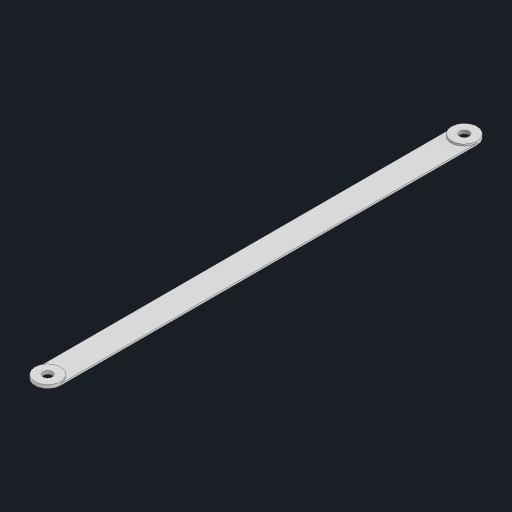
# Autodesk Inventor part: kozepso szalag2
Saved by Autodesk Inventor 2023 (Build 270158000, 158)
## iProperties
Created: 2022-11-11
Part Number: kozepso szalag2
Material: Generic
Document SubType Name: Modeling
Designer: gd1
Density: 1 g/cm^3
Appearance: Default
Mass: 4.10146 g
Surface Area: 82.9042 cm^2
Volume: 4.10146 cm^3
Author: gd1
Autodesk Inventor part; units mm, degrees
ref_plane "YZ Plane" through (0, 0, 0) normal (1, 0, 0) x (0, 1, 0)
ref_plane "XZ Plane" through (0, 0, 0) normal (0, 1, 0) x (-1, 0, 0)
ref_plane "XY Plane" through (0, 0, 0) normal (0, 0, 1) x (1, 0, 0)
sketch "Sketch1" plane through (0, 0, 0) normal (0, 1, 0) x (-1, 0, 0)
  circle A0 centre (0, 0) radius 2.75
  circle A1 centre (0, 0) radius 7.5
  circle A2 centre (0, -244.423) radius 2.75
  circle A3 centre (0, -244.423) radius 7.5
  line L0 (0, 7.5) -> (0, -251.923) construction
  line L1 (7.5, 0) -> (7.5, -244.423)
  line L2 (-7.5, 0) -> (-7.5, -244.423)
  dimension "d0" = 5.5
  dimension "d1" = 15
  dimension "d14" = 5.5
  dimension "d15" = 15
  dimension "d20" = 259.423
  constraints: 6 end point, 6 point on circle, 4 centre point, 3 coincident, 2 parallel, 2 tangent, 1 vertical
  measures "d0" diameter of A0
  measures "d1" diameter of A1
  measures "d14" diameter of A2
  measures "d15" diameter of A3
  measures "d20" distance of L0.end L0.start
extrude "Extrusion4" add sketch "Sketch1" along normal blind 1 contours L1 A3 L2 A1
extrude "Extrusion5" add sketch "Sketch1" along normal blind 2 contours A1 | A3
body "Solid2"
